Autodesk Inventor part; units mm, degrees
(part 6 of 13)
  line L1967 (3.6169, 37.0758) -> (2.4634, 37.0758)
  arc A1969 (2.4634, 37.0758) -> (2.4634, 36.9498) centre (2.4634, 37.0128) ccw
  line L1968 (3.6799, 37.0128) -> (3.6799, 37.1921)
  arc A1970 (3.6799, 37.1921) -> (3.5539, 37.1921) centre (3.6169, 37.1921) ccw
  line L1969 (3.5539, 37.1921) -> (3.5539, 37.0128)
  arc A1971 (3.5539, 37.0128) -> (3.6799, 37.0128) centre (3.6169, 37.0128) ccw
  line L1970 (3.6751, 37.2162) -> (3.4898, 37.6634)
  arc A1972 (3.4898, 37.6634) -> (3.3734, 37.6152) centre (3.4316, 37.6393) ccw
  line L1971 (3.3734, 37.6152) -> (3.5587, 37.168)
  arc A1973 (3.5587, 37.168) -> (3.6751, 37.2162) centre (3.6169, 37.1921) ccw
  line L1972 (3.4761, 37.6838) -> (3.1338, 38.0261)
  arc A1974 (3.1338, 38.0261) -> (3.0448, 37.9371) centre (3.0893, 37.9816) ccw
  line L1973 (3.0448, 37.9371) -> (3.3871, 37.5948)
  arc A1975 (3.3871, 37.5948) -> (3.4761, 37.6838) centre (3.4316, 37.6393) ccw
  line L1974 (3.1134, 38.0398) -> (2.6662, 38.2251)
  arc A1976 (2.6662, 38.2251) -> (2.618, 38.1087) centre (2.6421, 38.1669) ccw
  line L1975 (2.618, 38.1087) -> (3.0652, 37.9234)
  arc A1977 (3.0652, 37.9234) -> (3.1134, 38.0398) centre (3.0893, 37.9816) ccw
  line L1976 (2.6421, 38.2299) -> (2.4628, 38.2299)
  arc A1978 (2.4628, 38.2299) -> (2.4628, 38.1039) centre (2.4628, 38.1669) ccw
  line L1977 (2.4628, 38.1039) -> (2.6421, 38.1039)
  arc A1979 (2.6421, 38.1039) -> (2.6421, 38.2299) centre (2.6421, 38.1669) ccw
  line L1978 (2.3998, 38.1669) -> (2.3998, 37.0134)
  arc A1980 (2.3998, 37.0134) -> (2.5258, 37.0134) centre (2.4628, 37.0134) ccw
  line L1979 (2.5258, 37.0134) -> (2.5258, 38.1669)
  arc A1981 (2.5258, 38.1669) -> (2.3998, 38.1669) centre (2.4628, 38.1669) ccw
  line L1980 (2.4628, 37.0764) -> (2.337, 37.0764)
  arc A1982 (2.337, 37.0764) -> (2.337, 36.9504) centre (2.337, 37.0134) ccw
  line L1981 (2.337, 36.9504) -> (2.4628, 36.9504)
  arc A1983 (2.4628, 36.9504) -> (2.4628, 37.0764) centre (2.4628, 37.0134) ccw
  line L1982 (2.4, 37.0134) -> (2.4, 38.1669)
  arc A1984 (2.4, 38.1669) -> (2.274, 38.1669) centre (2.337, 38.1669) ccw
  line L1983 (2.274, 38.1669) -> (2.274, 37.0134)
  arc A1985 (2.274, 37.0134) -> (2.4, 37.0134) centre (2.337, 37.0134) ccw
  line L1984 (2.337, 38.2299) -> (2.1578, 38.2299)
  arc A1986 (2.1578, 38.2299) -> (2.1578, 38.1039) centre (2.1578, 38.1669) ccw
  line L1985 (2.1578, 38.1039) -> (2.337, 38.1039)
  arc A1987 (2.337, 38.1039) -> (2.337, 38.2299) centre (2.337, 38.1669) ccw
  line L1986 (2.1337, 38.2251) -> (1.6865, 38.0398)
  arc A1988 (1.6865, 38.0398) -> (1.7347, 37.9234) centre (1.7106, 37.9816) ccw
  line L1987 (1.7347, 37.9234) -> (2.1819, 38.1087)
  arc A1989 (2.1819, 38.1087) -> (2.1337, 38.2251) centre (2.1578, 38.1669) ccw
  line L1988 (1.6661, 38.0261) -> (1.3238, 37.6838)
  arc A1990 (1.3238, 37.6838) -> (1.4128, 37.5948) centre (1.3683, 37.6393) ccw
  line L1989 (1.4128, 37.5948) -> (1.7551, 37.9371)
  arc A1991 (1.7551, 37.9371) -> (1.6661, 38.0261) centre (1.7106, 37.9816) ccw
  line L1990 (1.3101, 37.6634) -> (1.1248, 37.2162)
  arc A1992 (1.1248, 37.2162) -> (1.2412, 37.168) centre (1.183, 37.1921) ccw
  line L1991 (1.2412, 37.168) -> (1.4265, 37.6152)
  arc A1993 (1.4265, 37.6152) -> (1.3101, 37.6634) centre (1.3683, 37.6393) ccw
  line L1992 (1.12, 37.1921) -> (1.12, 37.0128)
  arc A1994 (1.12, 37.0128) -> (1.246, 37.0128) centre (1.183, 37.0128) ccw
  line L1993 (1.246, 37.0128) -> (1.246, 37.1921)
  arc A1995 (1.246, 37.1921) -> (1.12, 37.1921) centre (1.183, 37.1921) ccw
  line L1994 (1.183, 36.9498) -> (2.3365, 36.9498)
  arc A1996 (2.3365, 36.9498) -> (2.3365, 37.0758) centre (2.3365, 37.0128) ccw
  line L1995 (2.3365, 37.0758) -> (1.183, 37.0758)
  arc A1997 (1.183, 37.0758) -> (1.183, 36.9498) centre (1.183, 37.0128) ccw
  line L1996 (2.2735, 37.0128) -> (2.2735, 36.887)
  arc A1998 (2.2735, 36.887) -> (2.3995, 36.887) centre (2.3365, 36.887) ccw
  line L1997 (2.3995, 36.887) -> (2.3995, 37.0128)
  arc A1999 (2.3995, 37.0128) -> (2.2735, 37.0128) centre (2.3365, 37.0128) ccw
  line L1998 (2.3365, 36.95) -> (1.183, 36.95)
  arc A2000 (1.183, 36.95) -> (1.183, 36.824) centre (1.183, 36.887) ccw
  line L1999 (1.183, 36.824) -> (2.3365, 36.824)
  arc A2001 (2.3365, 36.824) -> (2.3365, 36.95) centre (2.3365, 36.887) ccw
  line L2000 (1.12, 36.887) -> (1.12, 36.7078)
  arc A2002 (1.12, 36.7078) -> (1.246, 36.7078) centre (1.183, 36.7078) ccw
  line L2001 (1.246, 36.7078) -> (1.246, 36.887)
  arc A2003 (1.246, 36.887) -> (1.12, 36.887) centre (1.183, 36.887) ccw
  line L2002 (1.1248, 36.6837) -> (1.3101, 36.2365)
  arc A2004 (1.3101, 36.2365) -> (1.4265, 36.2847) centre (1.3683, 36.2606) ccw
  line L2003 (1.4265, 36.2847) -> (1.2412, 36.7319)
  arc A2005 (1.2412, 36.7319) -> (1.1248, 36.6837) centre (1.183, 36.7078) ccw
  line L2004 (1.3238, 36.2161) -> (1.6661, 35.8738)
  arc A2006 (1.6661, 35.8738) -> (1.7551, 35.9628) centre (1.7106, 35.9183) ccw
  line L2005 (1.7551, 35.9628) -> (1.4128, 36.3051)
  arc A2007 (1.4128, 36.3051) -> (1.3238, 36.2161) centre (1.3683, 36.2606) ccw
  line L2006 (1.6865, 35.8601) -> (2.1337, 35.6748)
  arc A2008 (2.1337, 35.6748) -> (2.1819, 35.7912) centre (2.1578, 35.733) ccw
  line L2007 (2.1819, 35.7912) -> (1.7347, 35.9765)
  arc A2009 (1.7347, 35.9765) -> (1.6865, 35.8601) centre (1.7106, 35.9183) ccw
  line L2008 (3.5783, 47.2281) -> (3.5783, 47.6718)
  arc A2010 (3.5783, 47.6718) -> (3.4523, 47.6718) centre (3.5153, 47.6718) ccw
  line L2009 (3.4523, 47.6718) -> (3.4523, 47.2281)
  arc A2011 (3.4523, 47.2281) -> (3.5783, 47.2281) centre (3.5153, 47.2281) ccw
  line L2010 (3.5735, 47.6959) -> (3.4037, 48.1059)
  arc A2012 (3.4037, 48.1059) -> (3.2873, 48.0577) centre (3.3455, 48.0818) ccw
  line L2011 (3.2873, 48.0577) -> (3.4571, 47.6477)
  arc A2013 (3.4571, 47.6477) -> (3.5735, 47.6959) centre (3.5153, 47.6718) ccw
  line L2012 (3.39, 48.1263) -> (3.0763, 48.44)
  arc A2014 (3.0763, 48.44) -> (2.9873, 48.351) centre (3.0318, 48.3955) ccw
  line L2013 (2.9873, 48.351) -> (3.301, 48.0373)
  arc A2015 (3.301, 48.0373) -> (3.39, 48.1263) centre (3.3455, 48.0818) ccw
  line L2014 (3.0559, 48.4537) -> (2.6459, 48.6235)
  arc A2016 (2.6459, 48.6235) -> (2.5977, 48.5071) centre (2.6218, 48.5653) ccw
  line L2015 (2.5977, 48.5071) -> (3.0077, 48.3373)
  arc A2017 (3.0077, 48.3373) -> (3.0559, 48.4537) centre (3.0318, 48.3955) ccw
  line L2016 (2.6218, 48.6283) -> (2.1781, 48.6283)
  arc A2018 (2.1781, 48.6283) -> (2.1781, 48.5023) centre (2.1781, 48.5653) ccw
  line L2017 (2.1781, 48.5023) -> (2.6218, 48.5023)
  arc A2019 (2.6218, 48.5023) -> (2.6218, 48.6283) centre (2.6218, 48.5653) ccw
  line L2018 (2.154, 48.6235) -> (1.744, 48.4537)
  arc A2020 (1.744, 48.4537) -> (1.7922, 48.3373) centre (1.7681, 48.3955) ccw
  line L2019 (1.7922, 48.3373) -> (2.2022, 48.5071)
  arc A2021 (2.2022, 48.5071) -> (2.154, 48.6235) centre (2.1781, 48.5653) ccw
  line L2020 (1.7236, 48.44) -> (1.4099, 48.1263)
  arc A2022 (1.4099, 48.1263) -> (1.4989, 48.0373) centre (1.4544, 48.0818) ccw
  line L2021 (1.4989, 48.0373) -> (1.8126, 48.351)
  arc A2023 (1.8126, 48.351) -> (1.7236, 48.44) centre (1.7681, 48.3955) ccw
  line L2022 (1.3962, 48.1059) -> (1.2264, 47.6959)
  arc A2024 (1.2264, 47.6959) -> (1.3428, 47.6477) centre (1.2846, 47.6718) ccw
  line L2023 (1.3428, 47.6477) -> (1.5126, 48.0577)
  arc A2025 (1.5126, 48.0577) -> (1.3962, 48.1059) centre (1.4544, 48.0818) ccw
  line L2024 (1.2216, 47.6718) -> (1.2216, 47.2281)
  arc A2026 (1.2216, 47.2281) -> (1.3476, 47.2281) centre (1.2846, 47.2281) ccw
  line L2025 (1.3476, 47.2281) -> (1.3476, 47.6718)
  arc A2027 (1.3476, 47.6718) -> (1.2216, 47.6718) centre (1.2846, 47.6718) ccw
  line L2026 (1.2264, 47.204) -> (1.3962, 46.794)
  arc A2028 (1.3962, 46.794) -> (1.5126, 46.8422) centre (1.4544, 46.8181) ccw
  line L2027 (1.5126, 46.8422) -> (1.3428, 47.2522)
  arc A2029 (1.3428, 47.2522) -> (1.2264, 47.204) centre (1.2846, 47.2281) ccw
  line L2028 (1.4099, 46.7736) -> (1.7236, 46.4599)
  arc A2030 (1.7236, 46.4599) -> (1.8126, 46.5489) centre (1.7681, 46.5044) ccw
  line L2029 (1.8126, 46.5489) -> (1.4989, 46.8626)
  arc A2031 (1.4989, 46.8626) -> (1.4099, 46.7736) centre (1.4544, 46.8181) ccw
  line L2030 (1.744, 46.4462) -> (2.154, 46.2764)
  arc A2032 (2.154, 46.2764) -> (2.2022, 46.3928) centre (2.1781, 46.3346) ccw
  line L2031 (2.2022, 46.3928) -> (1.7922, 46.5626)
  arc A2033 (1.7922, 46.5626) -> (1.744, 46.4462) centre (1.7681, 46.5044) ccw
  line L2032 (2.1781, 46.2716) -> (2.6218, 46.2716)
  arc A2034 (2.6218, 46.2716) -> (2.6218, 46.3976) centre (2.6218, 46.3346) ccw
  line L2033 (2.6218, 46.3976) -> (2.1781, 46.3976)
  arc A2035 (2.1781, 46.3976) -> (2.1781, 46.2716) centre (2.1781, 46.3346) ccw
  line L2034 (2.6459, 46.2764) -> (3.0559, 46.4462)
  arc A2036 (3.0559, 46.4462) -> (3.0077, 46.5626) centre (3.0318, 46.5044) ccw
  line L2035 (3.0077, 46.5626) -> (2.5977, 46.3928)
  arc A2037 (2.5977, 46.3928) -> (2.6459, 46.2764) centre (2.6218, 46.3346) ccw
  line L2036 (3.0763, 46.4599) -> (3.39, 46.7736)
  arc A2038 (3.39, 46.7736) -> (3.301, 46.8626) centre (3.3455, 46.8181) ccw
  line L2037 (3.301, 46.8626) -> (2.9873, 46.5489)
  arc A2039 (2.9873, 46.5489) -> (3.0763, 46.4599) centre (3.0318, 46.5044) ccw
  line L2038 (3.4037, 46.794) -> (3.5735, 47.204)
  arc A2040 (3.5735, 47.204) -> (3.4571, 47.2522) centre (3.5153, 47.2281) ccw
  line L2039 (3.4571, 47.2522) -> (3.2873, 46.8422)
  arc A2041 (3.2873, 46.8422) -> (3.4037, 46.794) centre (3.3455, 46.8181) ccw
  line L2040 (2.1578, 49.67) -> (2.337, 49.67)
  arc A2042 (2.337, 49.67) -> (2.337, 49.796) centre (2.337, 49.733) ccw
  line L2041 (2.337, 49.796) -> (2.1578, 49.796)
  arc A2043 (2.1578, 49.796) -> (2.1578, 49.67) centre (2.1578, 49.733) ccw
  line L2042 (2.4, 49.733) -> (2.4, 50.8865)
  arc A2044 (2.4, 50.8865) -> (2.274, 50.8865) centre (2.337, 50.8865) ccw
  line L2043 (2.274, 50.8865) -> (2.274, 49.733)
  arc A2045 (2.274, 49.733) -> (2.4, 49.733) centre (2.337, 49.733) ccw
  line L2044 (2.337, 50.8235) -> (2.4628, 50.8235)
  arc A2046 (2.4628, 50.8235) -> (2.4628, 50.9495) centre (2.4628, 50.8865) ccw
  line L2045 (2.4628, 50.9495) -> (2.337, 50.9495)
  arc A2047 (2.337, 50.9495) -> (2.337, 50.8235) centre (2.337, 50.8865) ccw
  line L2046 (2.3998, 50.8865) -> (2.3998, 49.733)
  arc A2048 (2.3998, 49.733) -> (2.5258, 49.733) centre (2.4628, 49.733) ccw
  line L2047 (2.5258, 49.733) -> (2.5258, 50.8865)
  arc A2049 (2.5258, 50.8865) -> (2.3998, 50.8865) centre (2.4628, 50.8865) ccw
  line L2048 (2.4628, 49.67) -> (2.6421, 49.67)
  arc A2050 (2.6421, 49.67) -> (2.6421, 49.796) centre (2.6421, 49.733) ccw
  line L2049 (2.6421, 49.796) -> (2.4628, 49.796)
  arc A2051 (2.4628, 49.796) -> (2.4628, 49.67) centre (2.4628, 49.733) ccw
  line L2050 (2.6662, 49.6748) -> (3.1134, 49.8601)
  arc A2052 (3.1134, 49.8601) -> (3.0652, 49.9765) centre (3.0893, 49.9183) ccw
  line L2051 (3.0652, 49.9765) -> (2.618, 49.7912)
  arc A2053 (2.618, 49.7912) -> (2.6662, 49.6748) centre (2.6421, 49.733) ccw
  line L2052 (3.1338, 49.8738) -> (3.4761, 50.2161)
  arc A2054 (3.4761, 50.2161) -> (3.3871, 50.3051) centre (3.4316, 50.2606) ccw
  line L2053 (3.3871, 50.3051) -> (3.0448, 49.9628)
  arc A2055 (3.0448, 49.9628) -> (3.1338, 49.8738) centre (3.0893, 49.9183) ccw
  line L2054 (3.4898, 50.2365) -> (3.6751, 50.6837)
  arc A2056 (3.6751, 50.6837) -> (3.5587, 50.7319) centre (3.6169, 50.7078) ccw
  line L2055 (3.5587, 50.7319) -> (3.3734, 50.2847)
  arc A2057 (3.3734, 50.2847) -> (3.4898, 50.2365) centre (3.4316, 50.2606) ccw
  line L2056 (3.6799, 50.7078) -> (3.6799, 50.887)
  arc A2058 (3.6799, 50.887) -> (3.5539, 50.887) centre (3.6169, 50.887) ccw
  line L2057 (3.5539, 50.887) -> (3.5539, 50.7078)
  arc A2059 (3.5539, 50.7078) -> (3.6799, 50.7078) centre (3.6169, 50.7078) ccw
  line L2058 (3.6169, 50.95) -> (2.4634, 50.95)
  arc A2060 (2.4634, 50.95) -> (2.4634, 50.824) centre (2.4634, 50.887) ccw
  line L2059 (2.4634, 50.824) -> (3.6169, 50.824)
  arc A2061 (3.6169, 50.824) -> (3.6169, 50.95) centre (3.6169, 50.887) ccw
  line L2060 (2.5264, 50.887) -> (2.5264, 51.0128)
  arc A2062 (2.5264, 51.0128) -> (2.4004, 51.0128) centre (2.4634, 51.0128) ccw
  line L2061 (2.4004, 51.0128) -> (2.4004, 50.887)
  arc A2063 (2.4004, 50.887) -> (2.5264, 50.887) centre (2.4634, 50.887) ccw
  line L2062 (2.4634, 50.9498) -> (3.6169, 50.9498)
  arc A2064 (3.6169, 50.9498) -> (3.6169, 51.0758) centre (3.6169, 51.0128) ccw
  line L2063 (3.6169, 51.0758) -> (2.4634, 51.0758)
  arc A2065 (2.4634, 51.0758) -> (2.4634, 50.9498) centre (2.4634, 51.0128) ccw
  line L2064 (3.6799, 51.0128) -> (3.6799, 51.1921)
  arc A2066 (3.6799, 51.1921) -> (3.5539, 51.1921) centre (3.6169, 51.1921) ccw
  line L2065 (3.5539, 51.1921) -> (3.5539, 51.0128)
  arc A2067 (3.5539, 51.0128) -> (3.6799, 51.0128) centre (3.6169, 51.0128) ccw
  line L2066 (3.6751, 51.2162) -> (3.4898, 51.6634)
  arc A2068 (3.4898, 51.6634) -> (3.3734, 51.6152) centre (3.4316, 51.6393) ccw
  line L2067 (3.3734, 51.6152) -> (3.5587, 51.168)
  arc A2069 (3.5587, 51.168) -> (3.6751, 51.2162) centre (3.6169, 51.1921) ccw
  line L2068 (3.4761, 51.6838) -> (3.1338, 52.0261)
  arc A2070 (3.1338, 52.0261) -> (3.0448, 51.9371) centre (3.0893, 51.9816) ccw
  line L2069 (3.0448, 51.9371) -> (3.3871, 51.5948)
  arc A2071 (3.3871, 51.5948) -> (3.4761, 51.6838) centre (3.4316, 51.6393) ccw
  line L2070 (3.1134, 52.0398) -> (2.6662, 52.2251)
  arc A2072 (2.6662, 52.2251) -> (2.618, 52.1087) centre (2.6421, 52.1669) ccw
  line L2071 (2.618, 52.1087) -> (3.0652, 51.9234)
  arc A2073 (3.0652, 51.9234) -> (3.1134, 52.0398) centre (3.0893, 51.9816) ccw
  line L2072 (2.6421, 52.2299) -> (2.4628, 52.2299)
  arc A2074 (2.4628, 52.2299) -> (2.4628, 52.1039) centre (2.4628, 52.1669) ccw
  line L2073 (2.4628, 52.1039) -> (2.6421, 52.1039)
  arc A2075 (2.6421, 52.1039) -> (2.6421, 52.2299) centre (2.6421, 52.1669) ccw
  line L2074 (2.3998, 52.1669) -> (2.3998, 51.0134)
  arc A2076 (2.3998, 51.0134) -> (2.5258, 51.0134) centre (2.4628, 51.0134) ccw
  line L2075 (2.5258, 51.0134) -> (2.5258, 52.1669)
  arc A2077 (2.5258, 52.1669) -> (2.3998, 52.1669) centre (2.4628, 52.1669) ccw
  line L2076 (2.4628, 51.0764) -> (2.337, 51.0764)
  arc A2078 (2.337, 51.0764) -> (2.337, 50.9504) centre (2.337, 51.0134) ccw
  line L2077 (2.337, 50.9504) -> (2.4628, 50.9504)
  arc A2079 (2.4628, 50.9504) -> (2.4628, 51.0764) centre (2.4628, 51.0134) ccw
  line L2078 (2.4, 51.0134) -> (2.4, 52.1669)
  arc A2080 (2.4, 52.1669) -> (2.274, 52.1669) centre (2.337, 52.1669) ccw
  line L2079 (2.274, 52.1669) -> (2.274, 51.0134)
  arc A2081 (2.274, 51.0134) -> (2.4, 51.0134) centre (2.337, 51.0134) ccw
  line L2080 (2.337, 52.2299) -> (2.1578, 52.2299)
  arc A2082 (2.1578, 52.2299) -> (2.1578, 52.1039) centre (2.1578, 52.1669) ccw
  line L2081 (2.1578, 52.1039) -> (2.337, 52.1039)
  arc A2083 (2.337, 52.1039) -> (2.337, 52.2299) centre (2.337, 52.1669) ccw
  line L2082 (2.1337, 52.2251) -> (1.6865, 52.0398)
  arc A2084 (1.6865, 52.0398) -> (1.7347, 51.9234) centre (1.7106, 51.9816) ccw
  line L2083 (1.7347, 51.9234) -> (2.1819, 52.1087)
  arc A2085 (2.1819, 52.1087) -> (2.1337, 52.2251) centre (2.1578, 52.1669) ccw
  line L2084 (1.6661, 52.0261) -> (1.3238, 51.6838)
  arc A2086 (1.3238, 51.6838) -> (1.4128, 51.5948) centre (1.3683, 51.6393) ccw
  line L2085 (1.4128, 51.5948) -> (1.7551, 51.9371)
  arc A2087 (1.7551, 51.9371) -> (1.6661, 52.0261) centre (1.7106, 51.9816) ccw
  line L2086 (1.3101, 51.6634) -> (1.1248, 51.2162)
  arc A2088 (1.1248, 51.2162) -> (1.2412, 51.168) centre (1.183, 51.1921) ccw
  line L2087 (1.2412, 51.168) -> (1.4265, 51.6152)
  arc A2089 (1.4265, 51.6152) -> (1.3101, 51.6634) centre (1.3683, 51.6393) ccw
  line L2088 (1.12, 51.1921) -> (1.12, 51.0128)
  arc A2090 (1.12, 51.0128) -> (1.246, 51.0128) centre (1.183, 51.0128) ccw
  line L2089 (1.246, 51.0128) -> (1.246, 51.1921)
  arc A2091 (1.246, 51.1921) -> (1.12, 51.1921) centre (1.183, 51.1921) ccw
  line L2090 (1.183, 50.9498) -> (2.3365, 50.9498)
  arc A2092 (2.3365, 50.9498) -> (2.3365, 51.0758) centre (2.3365, 51.0128) ccw
  line L2091 (2.3365, 51.0758) -> (1.183, 51.0758)
  arc A2093 (1.183, 51.0758) -> (1.183, 50.9498) centre (1.183, 51.0128) ccw
  line L2092 (2.2735, 51.0128) -> (2.2735, 50.887)
  arc A2094 (2.2735, 50.887) -> (2.3995, 50.887) centre (2.3365, 50.887) ccw
  line L2093 (2.3995, 50.887) -> (2.3995, 51.0128)
  arc A2095 (2.3995, 51.0128) -> (2.2735, 51.0128) centre (2.3365, 51.0128) ccw
  line L2094 (2.3365, 50.95) -> (1.183, 50.95)
  arc A2096 (1.183, 50.95) -> (1.183, 50.824) centre (1.183, 50.887) ccw
  line L2095 (1.183, 50.824) -> (2.3365, 50.824)
  arc A2097 (2.3365, 50.824) -> (2.3365, 50.95) centre (2.3365, 50.887) ccw
  line L2096 (1.12, 50.887) -> (1.12, 50.7078)
  arc A2098 (1.12, 50.7078) -> (1.246, 50.7078) centre (1.183, 50.7078) ccw
  line L2097 (1.246, 50.7078) -> (1.246, 50.887)
  arc A2099 (1.246, 50.887) -> (1.12, 50.887) centre (1.183, 50.887) ccw
  line L2098 (1.1248, 50.6837) -> (1.3101, 50.2365)
  arc A2100 (1.3101, 50.2365) -> (1.4265, 50.2847) centre (1.3683, 50.2606) ccw
  line L2099 (1.4265, 50.2847) -> (1.2412, 50.7319)
  arc A2101 (1.2412, 50.7319) -> (1.1248, 50.6837) centre (1.183, 50.7078) ccw
  line L2100 (1.3238, 50.2161) -> (1.6661, 49.8738)
  arc A2102 (1.6661, 49.8738) -> (1.7551, 49.9628) centre (1.7106, 49.9183) ccw
  line L2101 (1.7551, 49.9628) -> (1.4128, 50.3051)
  arc A2103 (1.4128, 50.3051) -> (1.3238, 50.2161) centre (1.3683, 50.2606) ccw
  line L2102 (1.6865, 49.8601) -> (2.1337, 49.6748)
  arc A2104 (2.1337, 49.6748) -> (2.1819, 49.7912) centre (2.1578, 49.733) ccw
  line L2103 (2.1819, 49.7912) -> (1.7347, 49.9765)
  arc A2105 (1.7347, 49.9765) -> (1.6865, 49.8601) centre (1.7106, 49.9183) ccw
  line L2104 (8.8392, 5.3883) -> (6.5607, 5.3883)
  arc A2106 (6.5607, 5.3883) -> (6.5607, 5.2623) centre (6.5607, 5.3253) ccw
  line L2105 (6.5607, 5.2623) -> (8.8392, 5.2623)
  arc A2107 (8.8392, 5.2623) -> (8.8392, 5.3883) centre (8.8392, 5.3253) ccw
  line L2106 (6.5162, 5.3698) -> (6.3901, 5.2437)
  arc A2108 (6.3901, 5.2437) -> (6.4791, 5.1547) centre (6.4346, 5.1992) ccw
  line L2107 (6.4791, 5.1547) -> (6.6052, 5.2808)
  arc A2109 (6.6052, 5.2808) -> (6.5162, 5.3698) centre (6.5607, 5.3253) ccw
  line L2108 (6.3716, 5.1992) -> (6.3716, 2.9207)
  arc A2110 (6.3716, 2.9207) -> (6.4976, 2.9207) centre (6.4346, 2.9207) ccw
  line L2109 (6.4976, 2.9207) -> (6.4976, 5.1992)
  arc A2111 (6.4976, 5.1992) -> (6.3716, 5.1992) centre (6.4346, 5.1992) ccw
  line L2110 (6.3901, 2.8762) -> (6.5162, 2.7501)
  arc A2112 (6.5162, 2.7501) -> (6.6052, 2.8391) centre (6.5607, 2.7946) ccw
  line L2111 (6.6052, 2.8391) -> (6.4791, 2.9652)
  arc A2113 (6.4791, 2.9652) -> (6.3901, 2.8762) centre (6.4346, 2.9207) ccw
  line L2112 (6.5607, 2.7316) -> (8.8392, 2.7316)
  arc A2114 (8.8392, 2.7316) -> (8.8392, 2.8576) centre (8.8392, 2.7946) ccw
  line L2113 (8.8392, 2.8576) -> (6.5607, 2.8576)
  arc A2115 (6.5607, 2.8576) -> (6.5607, 2.7316) centre (6.5607, 2.7946) ccw
  line L2114 (8.8837, 2.7501) -> (9.0098, 2.8762)
  arc A2116 (9.0098, 2.8762) -> (8.9208, 2.9652) centre (8.9653, 2.9207) ccw
  line L2115 (8.9208, 2.9652) -> (8.7947, 2.8391)
  arc A2117 (8.7947, 2.8391) -> (8.8837, 2.7501) centre (8.8392, 2.7946) ccw
  line L2116 (9.0283, 2.9207) -> (9.0283, 5.1992)
  arc A2118 (9.0283, 5.1992) -> (8.9023, 5.1992) centre (8.9653, 5.1992) ccw
  line L2117 (8.9023, 5.1992) -> (8.9023, 2.9207)
  arc A2119 (8.9023, 2.9207) -> (9.0283, 2.9207) centre (8.9653, 2.9207) ccw
  line L2118 (9.0098, 5.2437) -> (8.8837, 5.3698)
  arc A2120 (8.8837, 5.3698) -> (8.7947, 5.2808) centre (8.8392, 5.3253) ccw
  line L2119 (8.7947, 5.2808) -> (8.9208, 5.1547)
  arc A2121 (8.9208, 5.1547) -> (9.0098, 5.2437) centre (8.9653, 5.1992) ccw
  line L2120 (7.428, 7.71) -> (7.637, 7.71)
  arc A2122 (7.637, 7.71) -> (7.637, 7.836) centre (7.637, 7.773) ccw
  line L2121 (7.637, 7.836) -> (7.428, 7.836)
  arc A2123 (7.428, 7.836) -> (7.428, 7.71) centre (7.428, 7.773) ccw
  line L2122 (7.7, 7.773) -> (7.7, 9.0765)
  arc A2124 (7.7, 9.0765) -> (7.574, 9.0765) centre (7.637, 9.0765) ccw
  line L2123 (7.574, 9.0765) -> (7.574, 7.773)
  arc A2125 (7.574, 7.773) -> (7.7, 7.773) centre (7.637, 7.773) ccw
  line L2124 (7.637, 9.0135) -> (7.7628, 9.0135)
  arc A2126 (7.7628, 9.0135) -> (7.7628, 9.1395) centre (7.7628, 9.0765) ccw
  line L2125 (7.7628, 9.1395) -> (7.637, 9.1395)
  arc A2127 (7.637, 9.1395) -> (7.637, 9.0135) centre (7.637, 9.0765) ccw
  line L2126 (7.6998, 9.0765) -> (7.6998, 7.773)
  arc A2128 (7.6998, 7.773) -> (7.8258, 7.773) centre (7.7628, 7.773) ccw
  line L2127 (7.8258, 7.773) -> (7.8258, 9.0765)
  arc A2129 (7.8258, 9.0765) -> (7.6998, 9.0765) centre (7.7628, 9.0765) ccw
  line L2128 (7.7628, 7.71) -> (7.9719, 7.71)
  arc A2130 (7.9719, 7.71) -> (7.9719, 7.836) centre (7.9719, 7.773) ccw
  line L2129 (7.9719, 7.836) -> (7.7628, 7.836)
  arc A2131 (7.7628, 7.836) -> (7.7628, 7.71) centre (7.7628, 7.773) ccw
  line L2130 (7.996, 7.7148) -> (8.4984, 7.9229)
  arc A2132 (8.4984, 7.9229) -> (8.4502, 8.0393) centre (8.4743, 7.9811) ccw
  line L2131 (8.4502, 8.0393) -> (7.9478, 7.8312)
  arc A2133 (7.9478, 7.8312) -> (7.996, 7.7148) centre (7.9719, 7.773) ccw
  line L2132 (8.5188, 7.9366) -> (8.9033, 8.3211)
  arc A2134 (8.9033, 8.3211) -> (8.8143, 8.4101) centre (8.8588, 8.3656) ccw
  line L2133 (8.8143, 8.4101) -> (8.4298, 8.0256)
  arc A2135 (8.4298, 8.0256) -> (8.5188, 7.9366) centre (8.4743, 7.9811) ccw
  line L2134 (8.917, 8.3415) -> (9.1251, 8.8439)
  arc A2136 (9.1251, 8.8439) -> (9.0087, 8.8921) centre (9.0669, 8.868) ccw
  line L2135 (9.0087, 8.8921) -> (8.8006, 8.3897)
  arc A2137 (8.8006, 8.3897) -> (8.917, 8.3415) centre (8.8588, 8.3656) ccw
  line L2136 (9.1299, 8.868) -> (9.1299, 9.077)
  arc A2138 (9.1299, 9.077) -> (9.0039, 9.077) centre (9.0669, 9.077) ccw
  line L2137 (9.0039, 9.077) -> (9.0039, 8.868)
  arc A2139 (9.0039, 8.868) -> (9.1299, 8.868) centre (9.0669, 8.868) ccw
  line L2138 (9.0669, 9.14) -> (7.7634, 9.14)
  arc A2140 (7.7634, 9.14) -> (7.7634, 9.014) centre (7.7634, 9.077) ccw
  line L2139 (7.7634, 9.014) -> (9.0669, 9.014)
  arc A2141 (9.0669, 9.014) -> (9.0669, 9.14) centre (9.0669, 9.077) ccw
  line L2140 (7.8264, 9.077) -> (7.8264, 9.2028)
  arc A2142 (7.8264, 9.2028) -> (7.7004, 9.2028) centre (7.7634, 9.2028) ccw
  line L2141 (7.7004, 9.2028) -> (7.7004, 9.077)
  arc A2143 (7.7004, 9.077) -> (7.8264, 9.077) centre (7.7634, 9.077) ccw
  line L2142 (7.7634, 9.1398) -> (9.0669, 9.1398)
  arc A2144 (9.0669, 9.1398) -> (9.0669, 9.2658) centre (9.0669, 9.2028) ccw
  line L2143 (9.0669, 9.2658) -> (7.7634, 9.2658)
  arc A2145 (7.7634, 9.2658) -> (7.7634, 9.1398) centre (7.7634, 9.2028) ccw
  line L2144 (9.1299, 9.2028) -> (9.1299, 9.4119)
  arc A2146 (9.1299, 9.4119) -> (9.0039, 9.4119) centre (9.0669, 9.4119) ccw
  line L2145 (9.0039, 9.4119) -> (9.0039, 9.2028)
  arc A2147 (9.0039, 9.2028) -> (9.1299, 9.2028) centre (9.0669, 9.2028) ccw
  line L2146 (9.1251, 9.436) -> (8.917, 9.9384)
  arc A2148 (8.917, 9.9384) -> (8.8006, 9.8902) centre (8.8588, 9.9143) ccw
  line L2147 (8.8006, 9.8902) -> (9.0087, 9.3878)
  arc A2149 (9.0087, 9.3878) -> (9.1251, 9.436) centre (9.0669, 9.4119) ccw
  line L2148 (8.9033, 9.9588) -> (8.5188, 10.3433)
  arc A2150 (8.5188, 10.3433) -> (8.4298, 10.2543) centre (8.4743, 10.2988) ccw
  line L2149 (8.4298, 10.2543) -> (8.8143, 9.8698)
  arc A2151 (8.8143, 9.8698) -> (8.9033, 9.9588) centre (8.8588, 9.9143) ccw
  line L2150 (8.4984, 10.357) -> (7.996, 10.5651)
  arc A2152 (7.996, 10.5651) -> (7.9478, 10.4487) centre (7.9719, 10.5069) ccw
  line L2151 (7.9478, 10.4487) -> (8.4502, 10.2406)
  arc A2153 (8.4502, 10.2406) -> (8.4984, 10.357) centre (8.4743, 10.2988) ccw
  line L2152 (7.9719, 10.5699) -> (7.7628, 10.5699)
  arc A2154 (7.7628, 10.5699) -> (7.7628, 10.4439) centre (7.7628, 10.5069) ccw
  line L2153 (7.7628, 10.4439) -> (7.9719, 10.4439)
  arc A2155 (7.9719, 10.4439) -> (7.9719, 10.5699) centre (7.9719, 10.5069) ccw
  line L2154 (7.6998, 10.5069) -> (7.6998, 9.2034)
  arc A2156 (7.6998, 9.2034) -> (7.8258, 9.2034) centre (7.7628, 9.2034) ccw
  line L2155 (7.8258, 9.2034) -> (7.8258, 10.5069)
  arc A2157 (7.8258, 10.5069) -> (7.6998, 10.5069) centre (7.7628, 10.5069) ccw
  line L2156 (7.7628, 9.2664) -> (7.637, 9.2664)
  arc A2158 (7.637, 9.2664) -> (7.637, 9.1404) centre (7.637, 9.2034) ccw
  line L2157 (7.637, 9.1404) -> (7.7628, 9.1404)
  arc A2159 (7.7628, 9.1404) -> (7.7628, 9.2664) centre (7.7628, 9.2034) ccw
  line L2158 (7.7, 9.2034) -> (7.7, 10.5069)
  arc A2160 (7.7, 10.5069) -> (7.574, 10.5069) centre (7.637, 10.5069) ccw
  line L2159 (7.574, 10.5069) -> (7.574, 9.2034)
  arc A2161 (7.574, 9.2034) -> (7.7, 9.2034) centre (7.637, 9.2034) ccw
  line L2160 (7.637, 10.5699) -> (7.428, 10.5699)
  arc A2162 (7.428, 10.5699) -> (7.428, 10.4439) centre (7.428, 10.5069) ccw
  line L2161 (7.428, 10.4439) -> (7.637, 10.4439)
  arc A2163 (7.637, 10.4439) -> (7.637, 10.5699) centre (7.637, 10.5069) ccw
  line L2162 (7.4039, 10.5651) -> (6.9015, 10.357)
  arc A2164 (6.9015, 10.357) -> (6.9497, 10.2406) centre (6.9256, 10.2988) ccw
  line L2163 (6.9497, 10.2406) -> (7.4521, 10.4487)
  arc A2165 (7.4521, 10.4487) -> (7.4039, 10.5651) centre (7.428, 10.5069) ccw
  line L2164 (6.8811, 10.3433) -> (6.4966, 9.9588)
  arc A2166 (6.4966, 9.9588) -> (6.5856, 9.8698) centre (6.5411, 9.9143) ccw
  line L2165 (6.5856, 9.8698) -> (6.9701, 10.2543)
  arc A2167 (6.9701, 10.2543) -> (6.8811, 10.3433) centre (6.9256, 10.2988) ccw
  line L2166 (6.4829, 9.9384) -> (6.2748, 9.436)
  arc A2168 (6.2748, 9.436) -> (6.3912, 9.3878) centre (6.333, 9.4119) ccw
  line L2167 (6.3912, 9.3878) -> (6.5993, 9.8902)
  arc A2169 (6.5993, 9.8902) -> (6.4829, 9.9384) centre (6.5411, 9.9143) ccw
  line L2168 (6.27, 9.4119) -> (6.27, 9.2028)
  arc A2170 (6.27, 9.2028) -> (6.396, 9.2028) centre (6.333, 9.2028) ccw
  line L2169 (6.396, 9.2028) -> (6.396, 9.4119)
  arc A2171 (6.396, 9.4119) -> (6.27, 9.4119) centre (6.333, 9.4119) ccw
  line L2170 (6.333, 9.1398) -> (7.6365, 9.1398)
  arc A2172 (7.6365, 9.1398) -> (7.6365, 9.2658) centre (7.6365, 9.2028) ccw
  line L2171 (7.6365, 9.2658) -> (6.333, 9.2658)
  arc A2173 (6.333, 9.2658) -> (6.333, 9.1398) centre (6.333, 9.2028) ccw
  line L2172 (7.5735, 9.2028) -> (7.5735, 9.077)
  arc A2174 (7.5735, 9.077) -> (7.6995, 9.077) centre (7.6365, 9.077) ccw
  line L2173 (7.6995, 9.077) -> (7.6995, 9.2028)
  arc A2175 (7.6995, 9.2028) -> (7.5735, 9.2028) centre (7.6365, 9.2028) ccw
  line L2174 (7.6365, 9.14) -> (6.333, 9.14)
  arc A2176 (6.333, 9.14) -> (6.333, 9.014) centre (6.333, 9.077) ccw
  line L2175 (6.333, 9.014) -> (7.6365, 9.014)
  arc A2177 (7.6365, 9.014) -> (7.6365, 9.14) centre (7.6365, 9.077) ccw
  line L2176 (6.27, 9.077) -> (6.27, 8.868)
  arc A2178 (6.27, 8.868) -> (6.396, 8.868) centre (6.333, 8.868) ccw
  line L2177 (6.396, 8.868) -> (6.396, 9.077)
  arc A2179 (6.396, 9.077) -> (6.27, 9.077) centre (6.333, 9.077) ccw
  line L2178 (6.2748, 8.8439) -> (6.4829, 8.3415)
  arc A2180 (6.4829, 8.3415) -> (6.5993, 8.3897) centre (6.5411, 8.3656) ccw
  line L2179 (6.5993, 8.3897) -> (6.3912, 8.8921)
  arc A2181 (6.3912, 8.8921) -> (6.2748, 8.8439) centre (6.333, 8.868) ccw
  line L2180 (6.4966, 8.3211) -> (6.8811, 7.9366)
  arc A2182 (6.8811, 7.9366) -> (6.9701, 8.0256) centre (6.9256, 7.9811) ccw
  line L2181 (6.9701, 8.0256) -> (6.5856, 8.4101)
  arc A2183 (6.5856, 8.4101) -> (6.4966, 8.3211) centre (6.5411, 8.3656) ccw
  line L2182 (6.9015, 7.9229) -> (7.4039, 7.7148)
  arc A2184 (7.4039, 7.7148) -> (7.4521, 7.8312) centre (7.428, 7.773) ccw
  line L2183 (7.4521, 7.8312) -> (6.9497, 8.0393)
  arc A2185 (6.9497, 8.0393) -> (6.9015, 7.9229) centre (6.9256, 7.9811) ccw
  line L2184 (9.0283, 24.1282) -> (9.0283, 24.6317)
  arc A2186 (9.0283, 24.6317) -> (8.9023, 24.6317) centre (8.9653, 24.6317) ccw
  line L2185 (8.9023, 24.6317) -> (8.9023, 24.1282)
  arc A2187 (8.9023, 24.1282) -> (9.0283, 24.1282) centre (8.9653, 24.1282) ccw
  line L2186 (9.0235, 24.6558) -> (8.8309, 25.1208)
  arc A2188 (8.8309, 25.1208) -> (8.7145, 25.0726) centre (8.7727, 25.0967) ccw
  line L2187 (8.7145, 25.0726) -> (8.9071, 24.6076)
  arc A2189 (8.9071, 24.6076) -> (9.0235, 24.6558) centre (8.9653, 24.6317) ccw
  line L2188 (8.8172, 25.1412) -> (8.4612, 25.4972)
  arc A2190 (8.4612, 25.4972) -> (8.3722, 25.4082) centre (8.4167, 25.4527) ccw
  line L2189 (8.3722, 25.4082) -> (8.7282, 25.0522)
  arc A2191 (8.7282, 25.0522) -> (8.8172, 25.1412) centre (8.7727, 25.0967) ccw
  line L2190 (8.4408, 25.5109) -> (7.9758, 25.7035)
  arc A2192 (7.9758, 25.7035) -> (7.9276, 25.5871) centre (7.9517, 25.6453) ccw
  line L2191 (7.9276, 25.5871) -> (8.3926, 25.3945)
  arc A2193 (8.3926, 25.3945) -> (8.4408, 25.5109) centre (8.4167, 25.4527) ccw
  line L2192 (7.9517, 25.7083) -> (7.4482, 25.7083)
  arc A2194 (7.4482, 25.7083) -> (7.4482, 25.5823) centre (7.4482, 25.6453) ccw
  line L2193 (7.4482, 25.5823) -> (7.9517, 25.5823)
  arc A2195 (7.9517, 25.5823) -> (7.9517, 25.7083) centre (7.9517, 25.6453) ccw
  line L2194 (7.4241, 25.7035) -> (6.9591, 25.5109)
  arc A2196 (6.9591, 25.5109) -> (7.0073, 25.3945) centre (6.9832, 25.4527) ccw
  line L2195 (7.0073, 25.3945) -> (7.4723, 25.5871)
  arc A2197 (7.4723, 25.5871) -> (7.4241, 25.7035) centre (7.4482, 25.6453) ccw
  line L2196 (6.9387, 25.4972) -> (6.5827, 25.1412)
  arc A2198 (6.5827, 25.1412) -> (6.6717, 25.0522) centre (6.6272, 25.0967) ccw
  line L2197 (6.6717, 25.0522) -> (7.0277, 25.4082)
  arc A2199 (7.0277, 25.4082) -> (6.9387, 25.4972) centre (6.9832, 25.4527) ccw
  line L2198 (6.569, 25.1208) -> (6.3764, 24.6558)
  arc A2200 (6.3764, 24.6558) -> (6.4928, 24.6076) centre (6.4346, 24.6317) ccw
  line L2199 (6.4928, 24.6076) -> (6.6854, 25.0726)
  arc A2201 (6.6854, 25.0726) -> (6.569, 25.1208) centre (6.6272, 25.0967) ccw
  line L2200 (6.3716, 24.6317) -> (6.3716, 24.1282)
  arc A2202 (6.3716, 24.1282) -> (6.4976, 24.1282) centre (6.4346, 24.1282) ccw
  line L2201 (6.4976, 24.1282) -> (6.4976, 24.6317)
  arc A2203 (6.4976, 24.6317) -> (6.3716, 24.6317) centre (6.4346, 24.6317) ccw
  line L2202 (6.3764, 24.1041) -> (6.569, 23.6391)
  arc A2204 (6.569, 23.6391) -> (6.6854, 23.6873) centre (6.6272, 23.6632) ccw
  line L2203 (6.6854, 23.6873) -> (6.4928, 24.1523)
  arc A2205 (6.4928, 24.1523) -> (6.3764, 24.1041) centre (6.4346, 24.1282) ccw
  line L2204 (6.5827, 23.6187) -> (6.9387, 23.2627)
  arc A2206 (6.9387, 23.2627) -> (7.0277, 23.3517) centre (6.9832, 23.3072) ccw
  line L2205 (7.0277, 23.3517) -> (6.6717, 23.7077)
  arc A2207 (6.6717, 23.7077) -> (6.5827, 23.6187) centre (6.6272, 23.6632) ccw
  line L2206 (6.9591, 23.249) -> (7.4241, 23.0564)
  arc A2208 (7.4241, 23.0564) -> (7.4723, 23.1728) centre (7.4482, 23.1146) ccw
  line L2207 (7.4723, 23.1728) -> (7.0073, 23.3654)
  arc A2209 (7.0073, 23.3654) -> (6.9591, 23.249) centre (6.9832, 23.3072) ccw
  line L2208 (7.4482, 23.0516) -> (7.9517, 23.0516)
  arc A2210 (7.9517, 23.0516) -> (7.9517, 23.1776) centre (7.9517, 23.1146) ccw
  line L2209 (7.9517, 23.1776) -> (7.4482, 23.1776)
  arc A2211 (7.4482, 23.1776) -> (7.4482, 23.0516) centre (7.4482, 23.1146) ccw
  line L2210 (7.9758, 23.0564) -> (8.4408, 23.249)
  arc A2212 (8.4408, 23.249) -> (8.3926, 23.3654) centre (8.4167, 23.3072) ccw
  line L2211 (8.3926, 23.3654) -> (7.9276, 23.1728)
  arc A2213 (7.9276, 23.1728) -> (7.9758, 23.0564) centre (7.9517, 23.1146) ccw
  line L2212 (8.4612, 23.2627) -> (8.8172, 23.6187)
  arc A2214 (8.8172, 23.6187) -> (8.7282, 23.7077) centre (8.7727, 23.6632) ccw
  line L2213 (8.7282, 23.7077) -> (8.3722, 23.3517)
  arc A2215 (8.3722, 23.3517) -> (8.4612, 23.2627) centre (8.4167, 23.3072) ccw
  line L2214 (8.8309, 23.6391) -> (9.0235, 24.1041)
  arc A2216 (9.0235, 24.1041) -> (8.9071, 24.1523) centre (8.9653, 24.1282) ccw
  line L2215 (8.9071, 24.1523) -> (8.7145, 23.6873)
  arc A2217 (8.7145, 23.6873) -> (8.8309, 23.6391) centre (8.7727, 23.6632) ccw
  line L2216 (7.428, 28.03) -> (7.637, 28.03)
  arc A2218 (7.637, 28.03) -> (7.637, 28.156) centre (7.637, 28.093) ccw
  line L2217 (7.637, 28.156) -> (7.428, 28.156)
  arc A2219 (7.428, 28.156) -> (7.428, 28.03) centre (7.428, 28.093) ccw
  line L2218 (7.7, 28.093) -> (7.7, 29.3965)
  arc A2220 (7.7, 29.3965) -> (7.574, 29.3965) centre (7.637, 29.3965) ccw
  line L2219 (7.574, 29.3965) -> (7.574, 28.093)
  arc A2221 (7.574, 28.093) -> (7.7, 28.093) centre (7.637, 28.093) ccw
  line L2220 (7.637, 29.3335) -> (7.7628, 29.3335)
  arc A2222 (7.7628, 29.3335) -> (7.7628, 29.4595) centre (7.7628, 29.3965) ccw
  line L2221 (7.7628, 29.4595) -> (7.637, 29.4595)
  arc A2223 (7.637, 29.4595) -> (7.637, 29.3335) centre (7.637, 29.3965) ccw
  line L2222 (7.6998, 29.3965) -> (7.6998, 28.093)
  arc A2224 (7.6998, 28.093) -> (7.8258, 28.093) centre (7.7628, 28.093) ccw
  line L2223 (7.8258, 28.093) -> (7.8258, 29.3965)
  arc A2225 (7.8258, 29.3965) -> (7.6998, 29.3965) centre (7.7628, 29.3965) ccw
  line L2224 (7.7628, 28.03) -> (7.9719, 28.03)
  arc A2226 (7.9719, 28.03) -> (7.9719, 28.156) centre (7.9719, 28.093) ccw
  line L2225 (7.9719, 28.156) -> (7.7628, 28.156)
  arc A2227 (7.7628, 28.156) -> (7.7628, 28.03) centre (7.7628, 28.093) ccw
  line L2226 (7.996, 28.0348) -> (8.4984, 28.2429)
  arc A2228 (8.4984, 28.2429) -> (8.4502, 28.3593) centre (8.4743, 28.3011) ccw
  line L2227 (8.4502, 28.3593) -> (7.9478, 28.1512)
  arc A2229 (7.9478, 28.1512) -> (7.996, 28.0348) centre (7.9719, 28.093) ccw
  line L2228 (8.5188, 28.2566) -> (8.9033, 28.6411)
  arc A2230 (8.9033, 28.6411) -> (8.8143, 28.7301) centre (8.8588, 28.6856) ccw
  line L2229 (8.8143, 28.7301) -> (8.4298, 28.3456)
  arc A2231 (8.4298, 28.3456) -> (8.5188, 28.2566) centre (8.4743, 28.3011) ccw
  line L2230 (8.917, 28.6615) -> (9.1251, 29.1639)
  arc A2232 (9.1251, 29.1639) -> (9.0087, 29.2121) centre (9.0669, 29.188) ccw
  line L2231 (9.0087, 29.2121) -> (8.8006, 28.7097)
  arc A2233 (8.8006, 28.7097) -> (8.917, 28.6615) centre (8.8588, 28.6856) ccw
  line L2232 (9.1299, 29.188) -> (9.1299, 29.397)
  arc A2234 (9.1299, 29.397) -> (9.0039, 29.397) centre (9.0669, 29.397) ccw
  line L2233 (9.0039, 29.397) -> (9.0039, 29.188)
  arc A2235 (9.0039, 29.188) -> (9.1299, 29.188) centre (9.0669, 29.188) ccw
  line L2234 (9.0669, 29.46) -> (7.7634, 29.46)
  arc A2236 (7.7634, 29.46) -> (7.7634, 29.334) centre (7.7634, 29.397) ccw
  line L2235 (7.7634, 29.334) -> (9.0669, 29.334)
  arc A2237 (9.0669, 29.334) -> (9.0669, 29.46) centre (9.0669, 29.397) ccw
  line L2236 (7.8264, 29.397) -> (7.8264, 29.5228)
  arc A2238 (7.8264, 29.5228) -> (7.7004, 29.5228) centre (7.7634, 29.5228) ccw
  line L2237 (7.7004, 29.5228) -> (7.7004, 29.397)
  arc A2239 (7.7004, 29.397) -> (7.8264, 29.397) centre (7.7634, 29.397) ccw
  line L2238 (7.7634, 29.4598) -> (9.0669, 29.4598)
  arc A2240 (9.0669, 29.4598) -> (9.0669, 29.5858) centre (9.0669, 29.5228) ccw
  line L2239 (9.0669, 29.5858) -> (7.7634, 29.5858)
  arc A2241 (7.7634, 29.5858) -> (7.7634, 29.4598) centre (7.7634, 29.5228) ccw
  line L2240 (9.1299, 29.5228) -> (9.1299, 29.7319)
  arc A2242 (9.1299, 29.7319) -> (9.0039, 29.7319) centre (9.0669, 29.7319) ccw
  line L2241 (9.0039, 29.7319) -> (9.0039, 29.5228)
  arc A2243 (9.0039, 29.5228) -> (9.1299, 29.5228) centre (9.0669, 29.5228) ccw
  line L2242 (9.1251, 29.756) -> (8.917, 30.2584)
  arc A2244 (8.917, 30.2584) -> (8.8006, 30.2102) centre (8.8588, 30.2343) ccw
  line L2243 (8.8006, 30.2102) -> (9.0087, 29.7078)
  arc A2245 (9.0087, 29.7078) -> (9.1251, 29.756) centre (9.0669, 29.7319) ccw
  line L2244 (8.9033, 30.2788) -> (8.5188, 30.6633)
  arc A2246 (8.5188, 30.6633) -> (8.4298, 30.5743) centre (8.4743, 30.6188) ccw
  line L2245 (8.4298, 30.5743) -> (8.8143, 30.1898)
  arc A2247 (8.8143, 30.1898) -> (8.9033, 30.2788) centre (8.8588, 30.2343) ccw
  line L2246 (8.4984, 30.677) -> (7.996, 30.8851)
  arc A2248 (7.996, 30.8851) -> (7.9478, 30.7687) centre (7.9719, 30.8269) ccw
  line L2247 (7.9478, 30.7687) -> (8.4502, 30.5606)
  arc A2249 (8.4502, 30.5606) -> (8.4984, 30.677) centre (8.4743, 30.6188) ccw
  line L2248 (7.9719, 30.8899) -> (7.7628, 30.8899)
  arc A2250 (7.7628, 30.8899) -> (7.7628, 30.7639) centre (7.7628, 30.8269) ccw
  line L2249 (7.7628, 30.7639) -> (7.9719, 30.7639)
  arc A2251 (7.9719, 30.7639) -> (7.9719, 30.8899) centre (7.9719, 30.8269) ccw
  line L2250 (7.6998, 30.8269) -> (7.6998, 29.5234)
  arc A2252 (7.6998, 29.5234) -> (7.8258, 29.5234) centre (7.7628, 29.5234) ccw
  line L2251 (7.8258, 29.5234) -> (7.8258, 30.8269)
  arc A2253 (7.8258, 30.8269) -> (7.6998, 30.8269) centre (7.7628, 30.8269) ccw
  line L2252 (7.7628, 29.5864) -> (7.637, 29.5864)
  arc A2254 (7.637, 29.5864) -> (7.637, 29.4604) centre (7.637, 29.5234) ccw
  line L2253 (7.637, 29.4604) -> (7.7628, 29.4604)
  arc A2255 (7.7628, 29.4604) -> (7.7628, 29.5864) centre (7.7628, 29.5234) ccw
  line L2254 (7.7, 29.5234) -> (7.7, 30.8269)
  arc A2256 (7.7, 30.8269) -> (7.574, 30.8269) centre (7.637, 30.8269) ccw
  line L2255 (7.574, 30.8269) -> (7.574, 29.5234)
  arc A2257 (7.574, 29.5234) -> (7.7, 29.5234) centre (7.637, 29.5234) ccw
  line L2256 (7.637, 30.8899) -> (7.428, 30.8899)
  arc A2258 (7.428, 30.8899) -> (7.428, 30.7639) centre (7.428, 30.8269) ccw
  line L2257 (7.428, 30.7639) -> (7.637, 30.7639)
  arc A2259 (7.637, 30.7639) -> (7.637, 30.8899) centre (7.637, 30.8269) ccw
  line L2258 (7.4039, 30.8851) -> (6.9015, 30.677)
  arc A2260 (6.9015, 30.677) -> (6.9497, 30.5606) centre (6.9256, 30.6188) ccw
  line L2259 (6.9497, 30.5606) -> (7.4521, 30.7687)
  arc A2261 (7.4521, 30.7687) -> (7.4039, 30.8851) centre (7.428, 30.8269) ccw
  line L2260 (6.8811, 30.6633) -> (6.4966, 30.2788)
  arc A2262 (6.4966, 30.2788) -> (6.5856, 30.1898) centre (6.5411, 30.2343) ccw
  line L2261 (6.5856, 30.1898) -> (6.9701, 30.5743)
  arc A2263 (6.9701, 30.5743) -> (6.8811, 30.6633) centre (6.9256, 30.6188) ccw
  line L2262 (6.4829, 30.2584) -> (6.2748, 29.756)
  arc A2264 (6.2748, 29.756) -> (6.3912, 29.7078) centre (6.333, 29.7319) ccw
  line L2263 (6.3912, 29.7078) -> (6.5993, 30.2102)
  arc A2265 (6.5993, 30.2102) -> (6.4829, 30.2584) centre (6.5411, 30.2343) ccw
  line L2264 (6.27, 29.7319) -> (6.27, 29.5228)
  arc A2266 (6.27, 29.5228) -> (6.396, 29.5228) centre (6.333, 29.5228) ccw
  line L2265 (6.396, 29.5228) -> (6.396, 29.7319)
  arc A2267 (6.396, 29.7319) -> (6.27, 29.7319) centre (6.333, 29.7319) ccw
  line L2266 (6.333, 29.4598) -> (7.6365, 29.4598)
  arc A2268 (7.6365, 29.4598) -> (7.6365, 29.5858) centre (7.6365, 29.5228) ccw
  line L2267 (7.6365, 29.5858) -> (6.333, 29.5858)
  arc A2269 (6.333, 29.5858) -> (6.333, 29.4598) centre (6.333, 29.5228) ccw
  line L2268 (7.5735, 29.5228) -> (7.5735, 29.397)
  arc A2270 (7.5735, 29.397) -> (7.6995, 29.397) centre (7.6365, 29.397) ccw
  line L2269 (7.6995, 29.397) -> (7.6995, 29.5228)
  arc A2271 (7.6995, 29.5228) -> (7.5735, 29.5228) centre (7.6365, 29.5228) ccw
  line L2270 (7.6365, 29.46) -> (6.333, 29.46)
  arc A2272 (6.333, 29.46) -> (6.333, 29.334) centre (6.333, 29.397) ccw
  line L2271 (6.333, 29.334) -> (7.6365, 29.334)
  arc A2273 (7.6365, 29.334) -> (7.6365, 29.46) centre (7.6365, 29.397) ccw
  line L2272 (6.27, 29.397) -> (6.27, 29.188)
  arc A2274 (6.27, 29.188) -> (6.396, 29.188) centre (6.333, 29.188) ccw
  line L2273 (6.396, 29.188) -> (6.396, 29.397)
  arc A2275 (6.396, 29.397) -> (6.27, 29.397) centre (6.333, 29.397) ccw
  line L2274 (6.2748, 29.1639) -> (6.4829, 28.6615)
  arc A2276 (6.4829, 28.6615) -> (6.5993, 28.7097) centre (6.5411, 28.6856) ccw
  line L2275 (6.5993, 28.7097) -> (6.3912, 29.2121)
  arc A2277 (6.3912, 29.2121) -> (6.2748, 29.1639) centre (6.333, 29.188) ccw
  line L2276 (6.4966, 28.6411) -> (6.8811, 28.2566)
  arc A2278 (6.8811, 28.2566) -> (6.9701, 28.3456) centre (6.9256, 28.3011) ccw
  line L2277 (6.9701, 28.3456) -> (6.5856, 28.7301)
  arc A2279 (6.5856, 28.7301) -> (6.4966, 28.6411) centre (6.5411, 28.6856) ccw
  line L2278 (6.9015, 28.2429) -> (7.4039, 28.0348)
  arc A2280 (7.4039, 28.0348) -> (7.4521, 28.1512) centre (7.428, 28.093) ccw
  line L2279 (7.4521, 28.1512) -> (6.9497, 28.3593)
  arc A2281 (6.9497, 28.3593) -> (6.9015, 28.2429) centre (6.9256, 28.3011) ccw
  line L2280 (9.0283, 44.4482) -> (9.0283, 44.9517)
  arc A2282 (9.0283, 44.9517) -> (8.9023, 44.9517) centre (8.9653, 44.9517) ccw
  line L2281 (8.9023, 44.9517) -> (8.9023, 44.4482)
  arc A2283 (8.9023, 44.4482) -> (9.0283, 44.4482) centre (8.9653, 44.4482) ccw
  line L2282 (9.0235, 44.9758) -> (8.8309, 45.4408)
  arc A2284 (8.8309, 45.4408) -> (8.7145, 45.3926) centre (8.7727, 45.4167) ccw
  line L2283 (8.7145, 45.3926) -> (8.9071, 44.9276)
  arc A2285 (8.9071, 44.9276) -> (9.0235, 44.9758) centre (8.9653, 44.9517) ccw
  line L2284 (8.8172, 45.4612) -> (8.4612, 45.8172)
  arc A2286 (8.4612, 45.8172) -> (8.3722, 45.7282) centre (8.4167, 45.7727) ccw
  line L2285 (8.3722, 45.7282) -> (8.7282, 45.3722)
  arc A2287 (8.7282, 45.3722) -> (8.8172, 45.4612) centre (8.7727, 45.4167) ccw
  line L2286 (8.4408, 45.8309) -> (7.9758, 46.0235)
  arc A2288 (7.9758, 46.0235) -> (7.9276, 45.9071) centre (7.9517, 45.9653) ccw
  line L2287 (7.9276, 45.9071) -> (8.3926, 45.7145)
  arc A2289 (8.3926, 45.7145) -> (8.4408, 45.8309) centre (8.4167, 45.7727) ccw
  line L2288 (7.9517, 46.0283) -> (7.4482, 46.0283)
  arc A2290 (7.4482, 46.0283) -> (7.4482, 45.9023) centre (7.4482, 45.9653) ccw
  line L2289 (7.4482, 45.9023) -> (7.9517, 45.9023)
  arc A2291 (7.9517, 45.9023) -> (7.9517, 46.0283) centre (7.9517, 45.9653) ccw
  line L2290 (7.4241, 46.0235) -> (6.9591, 45.8309)
  arc A2292 (6.9591, 45.8309) -> (7.0073, 45.7145) centre (6.9832, 45.7727) ccw
  line L2291 (7.0073, 45.7145) -> (7.4723, 45.9071)
  arc A2293 (7.4723, 45.9071) -> (7.4241, 46.0235) centre (7.4482, 45.9653) ccw
  line L2292 (6.9387, 45.8172) -> (6.5827, 45.4612)
  arc A2294 (6.5827, 45.4612) -> (6.6717, 45.3722) centre (6.6272, 45.4167) ccw
  line L2293 (6.6717, 45.3722) -> (7.0277, 45.7282)
  arc A2295 (7.0277, 45.7282) -> (6.9387, 45.8172) centre (6.9832, 45.7727) ccw
  line L2294 (6.569, 45.4408) -> (6.3764, 44.9758)
  arc A2296 (6.3764, 44.9758) -> (6.4928, 44.9276) centre (6.4346, 44.9517) ccw
  line L2295 (6.4928, 44.9276) -> (6.6854, 45.3926)
  arc A2297 (6.6854, 45.3926) -> (6.569, 45.4408) centre (6.6272, 45.4167) ccw
  line L2296 (6.3716, 44.9517) -> (6.3716, 44.4482)
  arc A2298 (6.3716, 44.4482) -> (6.4976, 44.4482) centre (6.4346, 44.4482) ccw
  line L2297 (6.4976, 44.4482) -> (6.4976, 44.9517)
  arc A2299 (6.4976, 44.9517) -> (6.3716, 44.9517) centre (6.4346, 44.9517) ccw
  line L2298 (6.3764, 44.4241) -> (6.569, 43.9591)
  arc A2300 (6.569, 43.9591) -> (6.6854, 44.0073) centre (6.6272, 43.9832) ccw
  line L2299 (6.6854, 44.0073) -> (6.4928, 44.4723)
  arc A2301 (6.4928, 44.4723) -> (6.3764, 44.4241) centre (6.4346, 44.4482) ccw
  line L2300 (6.5827, 43.9387) -> (6.9387, 43.5827)
  arc A2302 (6.9387, 43.5827) -> (7.0277, 43.6717) centre (6.9832, 43.6272) ccw
  line L2301 (7.0277, 43.6717) -> (6.6717, 44.0277)
  arc A2303 (6.6717, 44.0277) -> (6.5827, 43.9387) centre (6.6272, 43.9832) ccw
  line L2302 (6.9591, 43.569) -> (7.4241, 43.3764)
  arc A2304 (7.4241, 43.3764) -> (7.4723, 43.4928) centre (7.4482, 43.4346) ccw
  line L2303 (7.4723, 43.4928) -> (7.0073, 43.6854)
  arc A2305 (7.0073, 43.6854) -> (6.9591, 43.569) centre (6.9832, 43.6272) ccw
  line L2304 (7.4482, 43.3716) -> (7.9517, 43.3716)
  arc A2306 (7.9517, 43.3716) -> (7.9517, 43.4976) centre (7.9517, 43.4346) ccw
  line L2305 (7.9517, 43.4976) -> (7.4482, 43.4976)
  arc A2307 (7.4482, 43.4976) -> (7.4482, 43.3716) centre (7.4482, 43.4346) ccw
  line L2306 (7.9758, 43.3764) -> (8.4408, 43.569)
  arc A2308 (8.4408, 43.569) -> (8.3926, 43.6854) centre (8.4167, 43.6272) ccw
  line L2307 (8.3926, 43.6854) -> (7.9276, 43.4928)
  arc A2309 (7.9276, 43.4928) -> (7.9758, 43.3764) centre (7.9517, 43.4346) ccw
  line L2308 (8.4612, 43.5827) -> (8.8172, 43.9387)
  arc A2310 (8.8172, 43.9387) -> (8.7282, 44.0277) centre (8.7727, 43.9832) ccw
  line L2309 (8.7282, 44.0277) -> (8.3722, 43.6717)
  arc A2311 (8.3722, 43.6717) -> (8.4612, 43.5827) centre (8.4167, 43.6272) ccw
  line L2310 (8.8309, 43.9591) -> (9.0235, 44.4241)
  arc A2312 (9.0235, 44.4241) -> (8.9071, 44.4723) centre (8.9653, 44.4482) ccw
  line L2311 (8.9071, 44.4723) -> (8.7145, 44.0073)
  arc A2313 (8.7145, 44.0073) -> (8.8309, 43.9591) centre (8.7727, 43.9832) ccw
  line L2312 (7.428, 48.35) -> (7.637, 48.35)
  arc A2314 (7.637, 48.35) -> (7.637, 48.476) centre (7.637, 48.413) ccw
  line L2313 (7.637, 48.476) -> (7.428, 48.476)
  arc A2315 (7.428, 48.476) -> (7.428, 48.35) centre (7.428, 48.413) ccw
  line L2314 (7.7, 48.413) -> (7.7, 49.7165)
  arc A2316 (7.7, 49.7165) -> (7.574, 49.7165) centre (7.637, 49.7165) ccw
  line L2315 (7.574, 49.7165) -> (7.574, 48.413)
  arc A2317 (7.574, 48.413) -> (7.7, 48.413) centre (7.637, 48.413) ccw
  line L2316 (7.637, 49.6535) -> (7.7628, 49.6535)
  arc A2318 (7.7628, 49.6535) -> (7.7628, 49.7795) centre (7.7628, 49.7165) ccw
  line L2317 (7.7628, 49.7795) -> (7.637, 49.7795)
  arc A2319 (7.637, 49.7795) -> (7.637, 49.6535) centre (7.637, 49.7165) ccw
  line L2318 (7.6998, 49.7165) -> (7.6998, 48.413)
  arc A2320 (7.6998, 48.413) -> (7.8258, 48.413) centre (7.7628, 48.413) ccw
  line L2319 (7.8258, 48.413) -> (7.8258, 49.7165)
  arc A2321 (7.8258, 49.7165) -> (7.6998, 49.7165) centre (7.7628, 49.7165) ccw
  line L2320 (7.7628, 48.35) -> (7.9719, 48.35)
  arc A2322 (7.9719, 48.35) -> (7.9719, 48.476) centre (7.9719, 48.413) ccw
  line L2321 (7.9719, 48.476) -> (7.7628, 48.476)
  arc A2323 (7.7628, 48.476) -> (7.7628, 48.35) centre (7.7628, 48.413) ccw
  line L2322 (7.996, 48.3548) -> (8.4984, 48.5629)
  arc A2324 (8.4984, 48.5629) -> (8.4502, 48.6793) centre (8.4743, 48.6211) ccw
  line L2323 (8.4502, 48.6793) -> (7.9478, 48.4712)
  arc A2325 (7.9478, 48.4712) -> (7.996, 48.3548) centre (7.9719, 48.413) ccw
  line L2324 (8.5188, 48.5766) -> (8.9033, 48.9611)
  arc A2326 (8.9033, 48.9611) -> (8.8143, 49.0501) centre (8.8588, 49.0056) ccw
  line L2325 (8.8143, 49.0501) -> (8.4298, 48.6656)
  arc A2327 (8.4298, 48.6656) -> (8.5188, 48.5766) centre (8.4743, 48.6211) ccw
  line L2326 (8.917, 48.9815) -> (9.1251, 49.4839)
  arc A2328 (9.1251, 49.4839) -> (9.0087, 49.5321) centre (9.0669, 49.508) ccw
  line L2327 (9.0087, 49.5321) -> (8.8006, 49.0297)
  arc A2329 (8.8006, 49.0297) -> (8.917, 48.9815) centre (8.8588, 49.0056) ccw
  line L2328 (9.1299, 49.508) -> (9.1299, 49.717)
  arc A2330 (9.1299, 49.717) -> (9.0039, 49.717) centre (9.0669, 49.717) ccw
  line L2329 (9.0039, 49.717) -> (9.0039, 49.508)
  arc A2331 (9.0039, 49.508) -> (9.1299, 49.508) centre (9.0669, 49.508) ccw
  line L2330 (9.0669, 49.78) -> (7.7634, 49.78)
  arc A2332 (7.7634, 49.78) -> (7.7634, 49.654) centre (7.7634, 49.717) ccw
  line L2331 (7.7634, 49.654) -> (9.0669, 49.654)
  arc A2333 (9.0669, 49.654) -> (9.0669, 49.78) centre (9.0669, 49.717) ccw
  line L2332 (7.8264, 49.717) -> (7.8264, 49.8428)
  arc A2334 (7.8264, 49.8428) -> (7.7004, 49.8428) centre (7.7634, 49.8428) ccw
  line L2333 (7.7004, 49.8428) -> (7.7004, 49.717)
  arc A2335 (7.7004, 49.717) -> (7.8264, 49.717) centre (7.7634, 49.717) ccw
  line L2334 (7.7634, 49.7798) -> (9.0669, 49.7798)
  arc A2336 (9.0669, 49.7798) -> (9.0669, 49.9058) centre (9.0669, 49.8428) ccw
  line L2335 (9.0669, 49.9058) -> (7.7634, 49.9058)
  arc A2337 (7.7634, 49.9058) -> (7.7634, 49.7798) centre (7.7634, 49.8428) ccw
  line L2336 (9.1299, 49.8428) -> (9.1299, 50.0519)
  arc A2338 (9.1299, 50.0519) -> (9.0039, 50.0519) centre (9.0669, 50.0519) ccw
  line L2337 (9.0039, 50.0519) -> (9.0039, 49.8428)
  arc A2339 (9.0039, 49.8428) -> (9.1299, 49.8428) centre (9.0669, 49.8428) ccw
  line L2338 (9.1251, 50.076) -> (8.917, 50.5784)
  arc A2340 (8.917, 50.5784) -> (8.8006, 50.5302) centre (8.8588, 50.5543) ccw
  line L2339 (8.8006, 50.5302) -> (9.0087, 50.0278)
  arc A2341 (9.0087, 50.0278) -> (9.1251, 50.076) centre (9.0669, 50.0519) ccw
  line L2340 (8.9033, 50.5988) -> (8.5188, 50.9833)
  arc A2342 (8.5188, 50.9833) -> (8.4298, 50.8943) centre (8.4743, 50.9388) ccw
  line L2341 (8.4298, 50.8943) -> (8.8143, 50.5098)
  arc A2343 (8.8143, 50.5098) -> (8.9033, 50.5988) centre (8.8588, 50.5543) ccw
  line L2342 (8.4984, 50.997) -> (7.996, 51.2051)
  arc A2344 (7.996, 51.2051) -> (7.9478, 51.0887) centre (7.9719, 51.1469) ccw
  line L2343 (7.9478, 51.0887) -> (8.4502, 50.8806)
  arc A2345 (8.4502, 50.8806) -> (8.4984, 50.997) centre (8.4743, 50.9388) ccw
  line L2344 (7.9719, 51.2099) -> (7.7628, 51.2099)
  arc A2346 (7.7628, 51.2099) -> (7.7628, 51.0839) centre (7.7628, 51.1469) ccw
  line L2345 (7.7628, 51.0839) -> (7.9719, 51.0839)
  arc A2347 (7.9719, 51.0839) -> (7.9719, 51.2099) centre (7.9719, 51.1469) ccw
  line L2346 (7.6998, 51.1469) -> (7.6998, 49.8434)
  arc A2348 (7.6998, 49.8434) -> (7.8258, 49.8434) centre (7.7628, 49.8434) ccw
  line L2347 (7.8258, 49.8434) -> (7.8258, 51.1469)
  arc A2349 (7.8258, 51.1469) -> (7.6998, 51.1469) centre (7.7628, 51.1469) ccw
  line L2348 (7.7628, 49.9064) -> (7.637, 49.9064)
  arc A2350 (7.637, 49.9064) -> (7.637, 49.7804) centre (7.637, 49.8434) ccw
  line L2349 (7.637, 49.7804) -> (7.7628, 49.7804)
  arc A2351 (7.7628, 49.7804) -> (7.7628, 49.9064) centre (7.7628, 49.8434) ccw
  line L2350 (7.7, 49.8434) -> (7.7, 51.1469)
  arc A2352 (7.7, 51.1469) -> (7.574, 51.1469) centre (7.637, 51.1469) ccw
  line L2351 (7.574, 51.1469) -> (7.574, 49.8434)
  arc A2353 (7.574, 49.8434) -> (7.7, 49.8434) centre (7.637, 49.8434) ccw
  line L2352 (7.637, 51.2099) -> (7.428, 51.2099)
  arc A2354 (7.428, 51.2099) -> (7.428, 51.0839) centre (7.428, 51.1469) ccw
  line L2353 (7.428, 51.0839) -> (7.637, 51.0839)
  arc A2355 (7.637, 51.0839) -> (7.637, 51.2099) centre (7.637, 51.1469) ccw
  line L2354 (7.4039, 51.2051) -> (6.9015, 50.997)